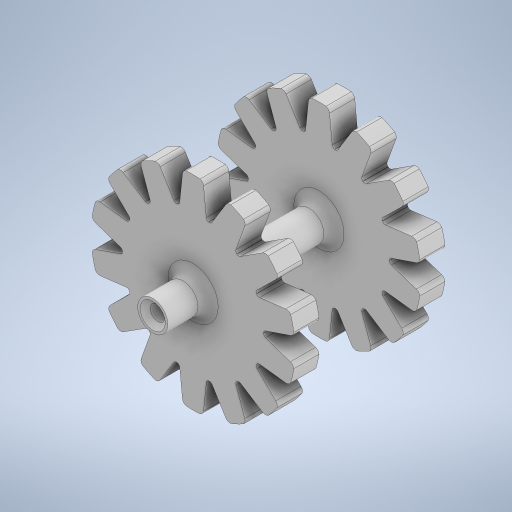
# Autodesk Inventor part: Zebatka
Saved by Autodesk Inventor 2024 (Build 280153000, 153)
## iProperties
Created: 2025-05-18
Part Number: Zebatka
Material: Ogólny
Document SubType Name: Modeling
Designer: Victoria
Density: 1 g/cm^3
Appearance: Domyślna
Author: Victoria
Autodesk Inventor part; units mm, degrees
ref_plane "YZ Plane" through (0, 0, 0) normal (1, 0, 0) x (0, 1, 0)
ref_plane "XZ Plane" through (0, 0, 0) normal (0, 1, 0) x (-1, 0, 0)
ref_plane "XY Plane" through (0, 0, 0) normal (0, 0, 1) x (1, 0, 0)
sketch "Szkic2" plane through (0, 0, 0) normal (0, 0, 1) x (1, 0, 0)
  circle A0 centre (0, 0) radius 20.25
  line L0 (0, 20.25) -> (1.0996, 20.25)
  line L1 (0, 20.25) -> (-1.0996, 20.25)
  circle A1 centre (0, 0) radius 14
  line L2 (-2.0941, 19.3545) -> (-2.6842, 13.7403)
  line L3 (-2, 20.25) -> (3.6452, 20.25) construction
  line L4 (2.0941, 19.3545) -> (2.6842, 13.7403)
  line L5 (2, 20.25) -> (7.6452, 20.25) construction
  arc A2 (-1.0996, 20.25) -> (-2.0941, 19.3545) centre (-1.0996, 19.25) ccw
  arc A3 (2.0941, 19.3545) -> (1.0996, 20.25) centre (1.0996, 19.25) ccw
  line L6 (-10.2844, 16.5292) -> (-8.3801, 11.2149)
  arc A4 (-9.7768, 17.7675) -> (-10.2844, 16.5292) centre (-9.343, 16.8666) ccw
  line L7 (-8.7861, 18.2446) -> (-9.7768, 17.7675)
  line L8 (-8.7861, 18.2446) -> (-7.7954, 18.7217)
  arc A5 (-6.5109, 18.3464) -> (-7.7954, 18.7217) centre (-7.3616, 17.8207) ccw
  line L9 (-6.5109, 18.3464) -> (-3.5433, 13.5442)
  line L10 (-16.4376, 10.4301) -> (-12.4161, 6.4683)
  arc A6 (-16.5177, 11.766) -> (-16.4376, 10.4301) centre (-15.7358, 11.1425) ccw
  line L11 (-15.8321, 12.6257) -> (-16.5177, 11.766)
  line L12 (-15.8321, 12.6257) -> (-15.1465, 13.4854)
  arc A7 (-13.8263, 13.7046) -> (-15.1465, 13.4854) centre (-14.3647, 12.8619) ccw
  line L13 (-13.8263, 13.7046) -> (-9.069, 10.6655)
  line L14 (-19.3353, 2.2652) -> (-13.9931, 0.4406)
  arc A8 (-19.987, 3.434) -> (-19.3353, 2.2652) centre (-19.012, 3.2115) ccw
  line L15 (-19.7423, 4.506) -> (-19.987, 3.434)
  line L16 (-19.7423, 4.506) -> (-19.4976, 5.5781)
  arc A9 (-18.4033, 6.3484) -> (-19.4976, 5.5781) centre (-18.5227, 5.3556) ccw
  line L17 (-18.4033, 6.3484) -> (-12.7985, 5.6744)
  line L18 (-18.4033, -6.3484) -> (-12.7985, -5.6744)
  arc A10 (-19.4976, -5.5781) -> (-18.4033, -6.3484) centre (-18.5227, -5.3556) ccw
  line L19 (-19.7423, -4.506) -> (-19.4976, -5.5781)
  line L20 (-19.7423, -4.506) -> (-19.987, -3.434)
  arc A11 (-19.3353, -2.2652) -> (-19.987, -3.434) centre (-19.012, -3.2115) ccw
  line L21 (-19.3353, -2.2652) -> (-13.9931, -0.4406)
  line L22 (-13.8263, -13.7046) -> (-9.069, -10.6655)
  arc A12 (-15.1465, -13.4854) -> (-13.8263, -13.7046) centre (-14.3647, -12.8619) ccw
  line L23 (-15.8321, -12.6257) -> (-15.1465, -13.4854)
  line L24 (-15.8321, -12.6257) -> (-16.5177, -11.766)
  arc A13 (-16.4376, -10.4301) -> (-16.5177, -11.766) centre (-15.7358, -11.1425) ccw
  line L25 (-16.4376, -10.4301) -> (-12.4161, -6.4683)
  line L26 (-6.5109, -18.3464) -> (-3.5433, -13.5442)
  arc A14 (-7.7954, -18.7217) -> (-6.5109, -18.3464) centre (-7.3616, -17.8207) ccw
  line L27 (-8.7861, -18.2446) -> (-7.7954, -18.7217)
  line L28 (-8.7861, -18.2446) -> (-9.7768, -17.7675)
  arc A15 (-10.2844, -16.5292) -> (-9.7768, -17.7675) centre (-9.343, -16.8666) ccw
  line L29 (-10.2844, -16.5292) -> (-8.3801, -11.2149)
  line L30 (2.0941, -19.3545) -> (2.6842, -13.7403)
  arc A16 (1.0996, -20.25) -> (2.0941, -19.3545) centre (1.0996, -19.25) ccw
  line L31 (0, -20.25) -> (1.0996, -20.25)
  line L32 (0, -20.25) -> (-1.0996, -20.25)
  arc A17 (-2.0941, -19.3545) -> (-1.0996, -20.25) centre (-1.0996, -19.25) ccw
  line L33 (-2.0941, -19.3545) -> (-2.6842, -13.7403)
  line L34 (10.2844, -16.5292) -> (8.3801, -11.2149)
  arc A18 (9.7768, -17.7675) -> (10.2844, -16.5292) centre (9.343, -16.8666) ccw
  line L35 (8.7861, -18.2446) -> (9.7768, -17.7675)
  line L36 (8.7861, -18.2446) -> (7.7954, -18.7217)
  arc A19 (6.5109, -18.3464) -> (7.7954, -18.7217) centre (7.3616, -17.8207) ccw
  line L37 (6.5109, -18.3464) -> (3.5433, -13.5442)
  line L38 (16.4376, -10.4301) -> (12.4161, -6.4683)
  arc A20 (16.5177, -11.766) -> (16.4376, -10.4301) centre (15.7358, -11.1425) ccw
  line L39 (15.8321, -12.6257) -> (16.5177, -11.766)
  line L40 (15.8321, -12.6257) -> (15.1465, -13.4854)
  arc A21 (13.8263, -13.7046) -> (15.1465, -13.4854) centre (14.3647, -12.8619) ccw
  line L41 (13.8263, -13.7046) -> (9.069, -10.6655)
  line L42 (19.3353, -2.2652) -> (13.9931, -0.4406)
  arc A22 (19.987, -3.434) -> (19.3353, -2.2652) centre (19.012, -3.2115) ccw
  line L43 (19.7423, -4.506) -> (19.987, -3.434)
  line L44 (19.7423, -4.506) -> (19.4976, -5.5781)
  arc A23 (18.4033, -6.3484) -> (19.4976, -5.5781) centre (18.5227, -5.3556) ccw
  line L45 (18.4033, -6.3484) -> (12.7985, -5.6744)
  line L46 (18.4033, 6.3484) -> (12.7985, 5.6744)
  arc A24 (19.4976, 5.5781) -> (18.4033, 6.3484) centre (18.5227, 5.3556) ccw
  line L47 (19.7423, 4.506) -> (19.4976, 5.5781)
  line L48 (19.7423, 4.506) -> (19.987, 3.434)
  arc A25 (19.3353, 2.2652) -> (19.987, 3.434) centre (19.012, 3.2115) ccw
  line L49 (19.3353, 2.2652) -> (13.9931, 0.4406)
  line L50 (13.8263, 13.7046) -> (9.069, 10.6655)
  arc A26 (15.1465, 13.4854) -> (13.8263, 13.7046) centre (14.3647, 12.8619) ccw
  line L51 (15.8321, 12.6257) -> (15.1465, 13.4854)
  line L52 (15.8321, 12.6257) -> (16.5177, 11.766)
  arc A27 (16.4376, 10.4301) -> (16.5177, 11.766) centre (15.7358, 11.1425) ccw
  line L53 (16.4376, 10.4301) -> (12.4161, 6.4683)
  line L54 (6.5109, 18.3464) -> (3.5433, 13.5442)
  arc A28 (7.7954, 18.7217) -> (6.5109, 18.3464) centre (7.3616, 17.8207) ccw
  line L55 (8.7861, 18.2446) -> (7.7954, 18.7217)
  line L56 (8.7861, 18.2446) -> (9.7768, 17.7675)
  arc A29 (10.2844, 16.5292) -> (9.7768, 17.7675) centre (9.343, 16.8666) ccw
  line L57 (10.2844, 16.5292) -> (8.3801, 11.2149)
  circle A30 centre (0, 0) radius 1.5
  point P0 (-10.5881, 17.3769)
  point P1 (-6.9842, 19.1124)
  point P2 (-17.0791, 11.062)
  point P3 (-14.5851, 14.1893)
  point P4 (-20.1873, 2.5562)
  point P5 (-19.2972, 6.4559)
  point P6 (-19.2972, -6.4559)
  point P7 (-20.1873, -2.5562)
  point P8 (-14.5851, -14.1893)
  point P9 (-17.0791, -11.062)
  point P10 (-6.9842, -19.1124)
  point P11 (-10.5881, -17.3769)
  point P12 (2, -20.25)
  point P13 (-2, -20.25)
  point P14 (10.5881, -17.3769)
  point P15 (6.9842, -19.1124)
  point P16 (17.0791, -11.062)
  point P17 (14.5851, -14.1893)
  point P18 (20.1873, -2.5562)
  point P19 (19.2972, -6.4559)
  point P20 (19.2972, 6.4559)
  point P21 (20.1873, 2.5562)
  point P22 (14.5851, 14.1893)
  point P23 (17.0791, 11.062)
  point P24 (6.9842, 19.1124)
  point P25 (10.5881, 17.3769)
  point P26 (-14.9152, 13.6967)
  point P27 (-16.6722, 11.4934)
  point P28 (-19.3809, 5.8688)
  point P29 (-20.008, 3.1214)
  point P30 (-20.008, -3.1214)
  point P31 (-19.3809, -5.8688)
  point P32 (-16.6722, -11.4934)
  point P33 (-14.9152, -13.6967)
  point P34 (-10.0343, -17.589)
  point P35 (-7.4954, -18.8118)
  point P36 (-1.409, -20.2009)
  point P37 (1.409, -20.2009)
  point P38 (7.4954, -18.8118)
  point P39 (10.0343, -17.589)
  point P40 (14.9152, -13.6967)
  point P41 (16.6722, -11.4934)
  point P42 (19.3809, -5.8688)
  point P43 (20.008, -3.1214)
  point P44 (20.008, 3.1214)
  point P45 (19.3809, 5.8688)
  point P46 (16.6722, 11.4934)
  point P47 (14.9152, 13.6967)
  point P48 (10.0343, 17.589)
  point P49 (7.4954, 18.8118)
  point P50 (1.409, 20.2009)
  point P51 (-1.409, 20.2009)
  point P52 (-7.4954, 18.8118)
  point P53 (-10.0343, 17.589)
  dimension "d14" = 40.5
  dimension "d17" = 6.25
  dimension "d15" = 2
  dimension "d16" = 2
  dimension "d18" = 264
  dimension "d19" = 84
  dimension "d20" = 1
  dimension "d23" = 360
  dimension "d25" = 3
  constraints: 116 end point, 70 point on line, 56 point on circle, 29 centre point, 4 horizontal, 4 tangent, 2 coincident, 2 equal length, 1 equal radius, 246 other
  measures "d15" distance of L0.start L5.start
  measures "d16" distance of L0.start L3.start
  measures "d19" angle of L4 L5
  measures "d20" radius of A2
  measures "d25" diameter of A30
extrude "Wyciągnięcie proste2" add sketch "Szkic2" along normal blind 5 contours A25 L49 A1 L46 A24 A0 | A0 A23 L45 A1 L42 A22 | A1 | A27 L53 A1 L50 A26 A0 | A0 A21 L41 A1 L38 A20 | A29 L57 A1 L54 A28 A0 | A0 A19 L37 A1 L34 A18 | A1 L2 A2 A0 A3 L4 | L30 A16 A0 A17 L33 A1 | A1 L6 A4 A0 A5 L9 | L26 A14 A0 A15 L29 A1 | A1 L10 A6 A0 A7 L13 | L22 A12 A0 A13 L25 A1 | A1 L14 A8 A0 A9 L17 | L18 A10 A0 A11 L21 A1
fillet "Zaokrąglenie1" radius 0.6 28 edges at (-13.9931, 0.4406, 2.5) (-13.9931, -0.4406, 2.5) (-12.7985, -5.6744, 2.5) (-12.4161, -6.4683, 2.5) (-8.3801, -11.2149, 2.5) (-9.069, -10.6655, 2.5) (-2.6842, -13.7403, 2.5) (-3.5433, -13.5442, 2.5) (3.5433, -13.5442, 2.5) (2.6842, -13.7403, 2.5) (9.069, -10.6655, 2.5) (8.3801, -11.2149, 2.5) (12.7985, -5.6744, 2.5) (12.4161, -6.4683, 2.5) (13.9931, 0.4406, 2.5) (13.9931, -0.4406, 2.5) (12.7985, 5.6744, 2.5) (12.4161, 6.4683, 2.5) (8.3801, 11.2149, 2.5) (9.069, 10.6655, 2.5) (2.6842, 13.7403, 2.5) (3.5433, 13.5442, 2.5) (-3.5433, 13.5442, 2.5) (-2.6842, 13.7403, 2.5) (-9.069, 10.6655, 2.5) (-8.3801, 11.2149, 2.5) (-12.7985, 5.6744, 2.5) (-12.4161, 6.4683, 2.5)
sketch "Szkic3" plane through (0, 0, 5) normal (0, 0, 1) x (1, 0, 0)
  circle A0 centre (0, 0) radius 1.5 projected
  circle A1 centre (0, 0) radius 3
  dimension "d29" = 6
  constraints: 1 centre point, 1 coincident
  measures "d29" diameter of A1
extrude "Wyciągnięcie proste3" add sketch "Szkic3" along normal blind 20 and the other way blind 8
sketch "Szkic4" plane through (0, 0, 25) normal (0, 0, 1) x (1, 0, 0)
  circle A0 centre (0, 0) radius 3 projected
  arc A1 (-13.8263, 13.7046) -> (-14.9152, 13.6967) centre (-14.3647, 12.8619) ccw projected
  arc A2 (-14.9152, 13.6967) -> (-16.6722, 11.4934) centre (0, 0) ccw projected
  arc A3 (-16.6722, 11.4934) -> (-16.4376, 10.4301) centre (-15.7358, 11.1425) ccw projected
  line L0 (-16.4376, 10.4301) -> (-12.727, 6.7746) projected
  arc A4 (-12.6078, 6.0863) -> (-12.727, 6.7746) centre (-13.1481, 6.3472) ccw projected
  arc A5 (-12.6078, 6.0863) -> (-12.6193, 6.0624) centre (0, 0) ccw projected
  arc A6 (-13.2318, 5.7265) -> (-12.6193, 6.0624) centre (-13.1602, 6.3222) ccw projected
  line L1 (-13.2318, 5.7265) -> (-18.4033, 6.3484) projected
  arc A7 (-18.4033, 6.3484) -> (-19.3809, 5.8688) centre (-18.5227, 5.3556) ccw projected
  arc A8 (-19.3809, 5.8688) -> (-20.008, 3.1214) centre (0, 0) ccw projected
  arc A9 (-20.008, 3.1214) -> (-19.3353, 2.2652) centre (-19.012, 3.2115) ccw projected
  line L2 (-19.3353, 2.2652) -> (-14.4061, 0.5817) projected
  arc A10 (-14, 0.0133) -> (-14.4061, 0.5817) centre (-14.6, 0.0139) ccw projected
  arc A11 (-14, 0.0133) -> (-14, -0.0133) centre (0, 0) ccw projected
  arc A12 (-14.4061, -0.5817) -> (-14, -0.0133) centre (-14.6, -0.0139) ccw projected
  line L3 (-14.4061, -0.5817) -> (-19.3353, -2.2652) projected
  arc A13 (-19.3353, -2.2652) -> (-20.008, -3.1214) centre (-19.012, -3.2115) ccw projected
  arc A14 (-20.008, -3.1214) -> (-19.3809, -5.8688) centre (0, 0) ccw projected
  arc A15 (-19.3809, -5.8688) -> (-18.4033, -6.3484) centre (-18.5227, -5.3556) ccw projected
  line L4 (-18.4033, -6.3484) -> (-13.2318, -5.7265) projected
  arc A16 (-12.6193, -6.0624) -> (-13.2318, -5.7265) centre (-13.1602, -6.3222) ccw projected
  arc A17 (-12.6193, -6.0624) -> (-12.6078, -6.0863) centre (0, 0) ccw projected
  arc A18 (-12.727, -6.7746) -> (-12.6078, -6.0863) centre (-13.1481, -6.3472) ccw projected
  line L5 (-12.727, -6.7746) -> (-16.4376, -10.4301) projected
  arc A19 (-16.4376, -10.4301) -> (-16.6722, -11.4934) centre (-15.7358, -11.1425) ccw projected
  arc A20 (-16.6722, -11.4934) -> (-14.9152, -13.6967) centre (0, 0) ccw projected
  arc A21 (-14.9152, -13.6967) -> (-13.8263, -13.7046) centre (-14.3647, -12.8619) ccw projected
  line L6 (-13.8263, -13.7046) -> (-9.4368, -10.9005) projected
  arc A22 (-8.7392, -10.9374) -> (-9.4368, -10.9005) centre (-9.1138, -11.4061) ccw projected
  arc A23 (-8.7392, -10.9374) -> (-8.7185, -10.9539) centre (0, 0) ccw projected
  arc A24 (-8.5273, -11.6258) -> (-8.7185, -10.9539) centre (-9.0921, -11.4234) ccw projected
  line L7 (-8.5273, -11.6258) -> (-10.2844, -16.5292) projected
  arc A25 (-10.2844, -16.5292) -> (-10.0343, -17.589) centre (-9.343, -16.8666) ccw projected
  arc A26 (-10.0343, -17.589) -> (-7.4954, -18.8118) centre (0, 0) ccw projected
  arc A27 (-7.4954, -18.8118) -> (-6.5109, -18.3464) centre (-7.3616, -17.8207) ccw projected
  line L8 (-6.5109, -18.3464) -> (-3.7727, -13.9154) projected
  arc A28 (-3.1282, -13.646) -> (-3.7727, -13.9154) centre (-3.2623, -14.2309) ccw projected
  arc A29 (-3.1282, -13.646) -> (-3.1023, -13.6519) centre (0, 0) ccw projected
  arc A30 (-2.6386, -14.1743) -> (-3.1023, -13.6519) centre (-3.2353, -14.237) ccw projected
  line L9 (-2.6386, -14.1743) -> (-2.0941, -19.3545) projected
  arc A31 (-2.0941, -19.3545) -> (-1.409, -20.2009) centre (-1.0996, -19.25) ccw projected
  arc A32 (-1.409, -20.2009) -> (1.409, -20.2009) centre (0, 0) ccw projected
  arc A33 (1.409, -20.2009) -> (2.0941, -19.3545) centre (1.0996, -19.25) ccw projected
  line L10 (2.0941, -19.3545) -> (2.6386, -14.1743) projected
  arc A34 (3.1023, -13.6519) -> (2.6386, -14.1743) centre (3.2353, -14.237) ccw projected
  arc A35 (3.1023, -13.6519) -> (3.1282, -13.646) centre (0, 0) ccw projected
  arc A36 (3.7727, -13.9154) -> (3.1282, -13.646) centre (3.2623, -14.2309) ccw projected
  line L11 (3.7727, -13.9154) -> (6.5109, -18.3464) projected
  arc A37 (6.5109, -18.3464) -> (7.4954, -18.8118) centre (7.3616, -17.8207) ccw projected
  arc A38 (7.4954, -18.8118) -> (10.0343, -17.589) centre (0, 0) ccw projected
  arc A39 (10.0343, -17.589) -> (10.2844, -16.5292) centre (9.343, -16.8666) ccw projected
  line L12 (10.2844, -16.5292) -> (8.5273, -11.6258) projected
  arc A40 (8.7185, -10.9539) -> (8.5273, -11.6258) centre (9.0921, -11.4234) ccw projected
  arc A41 (8.7185, -10.9539) -> (8.7392, -10.9374) centre (0, 0) ccw projected
  arc A42 (9.4368, -10.9005) -> (8.7392, -10.9374) centre (9.1138, -11.4061) ccw projected
  line L13 (9.4368, -10.9005) -> (13.8263, -13.7046) projected
  arc A43 (13.8263, -13.7046) -> (14.9152, -13.6967) centre (14.3647, -12.8619) ccw projected
  arc A44 (14.9152, -13.6967) -> (16.6722, -11.4934) centre (0, 0) ccw projected
  arc A45 (16.6722, -11.4934) -> (16.4376, -10.4301) centre (15.7358, -11.1425) ccw projected
  line L14 (16.4376, -10.4301) -> (12.727, -6.7746) projected
  arc A46 (12.6078, -6.0863) -> (12.727, -6.7746) centre (13.1481, -6.3472) ccw projected
  arc A47 (12.6078, -6.0863) -> (12.6193, -6.0624) centre (0, 0) ccw projected
  arc A48 (13.2318, -5.7265) -> (12.6193, -6.0624) centre (13.1602, -6.3222) ccw projected
  line L15 (13.2318, -5.7265) -> (18.4033, -6.3484) projected
  arc A49 (18.4033, -6.3484) -> (19.3809, -5.8688) centre (18.5227, -5.3556) ccw projected
  arc A50 (19.3809, -5.8688) -> (20.008, -3.1214) centre (0, 0) ccw projected
  arc A51 (20.008, -3.1214) -> (19.3353, -2.2652) centre (19.012, -3.2115) ccw projected
  line L16 (19.3353, -2.2652) -> (14.4061, -0.5817) projected
  arc A52 (14, -0.0133) -> (14.4061, -0.5817) centre (14.6, -0.0139) ccw projected
  arc A53 (14, -0.0133) -> (14, 0.0133) centre (0, 0) ccw projected
  arc A54 (14.4061, 0.5817) -> (14, 0.0133) centre (14.6, 0.0139) ccw projected
  line L17 (14.4061, 0.5817) -> (19.3353, 2.2652) projected
  arc A55 (19.3353, 2.2652) -> (20.008, 3.1214) centre (19.012, 3.2115) ccw projected
  arc A56 (20.008, 3.1214) -> (19.3809, 5.8688) centre (0, 0) ccw projected
  arc A57 (19.3809, 5.8688) -> (18.4033, 6.3484) centre (18.5227, 5.3556) ccw projected
  line L18 (18.4033, 6.3484) -> (13.2318, 5.7265) projected
  arc A58 (12.6193, 6.0624) -> (13.2318, 5.7265) centre (13.1602, 6.3222) ccw projected
  arc A59 (12.6193, 6.0624) -> (12.6078, 6.0863) centre (0, 0) ccw projected
  arc A60 (12.727, 6.7746) -> (12.6078, 6.0863) centre (13.1481, 6.3472) ccw projected
  line L19 (12.727, 6.7746) -> (16.4376, 10.4301) projected
  arc A61 (16.4376, 10.4301) -> (16.6722, 11.4934) centre (15.7358, 11.1425) ccw projected
  arc A62 (16.6722, 11.4934) -> (14.9152, 13.6967) centre (0, 0) ccw projected
  arc A63 (14.9152, 13.6967) -> (13.8263, 13.7046) centre (14.3647, 12.8619) ccw projected
  line L20 (13.8263, 13.7046) -> (9.4368, 10.9005) projected
  arc A64 (8.7392, 10.9374) -> (9.4368, 10.9005) centre (9.1138, 11.4061) ccw projected
  arc A65 (8.7392, 10.9374) -> (8.7185, 10.9539) centre (0, 0) ccw projected
  arc A66 (8.5273, 11.6258) -> (8.7185, 10.9539) centre (9.0921, 11.4234) ccw projected
  line L21 (8.5273, 11.6258) -> (10.2844, 16.5292) projected
  arc A67 (10.2844, 16.5292) -> (10.0343, 17.589) centre (9.343, 16.8666) ccw projected
  arc A68 (10.0343, 17.589) -> (7.4954, 18.8118) centre (0, 0) ccw projected
  arc A69 (7.4954, 18.8118) -> (6.5109, 18.3464) centre (7.3616, 17.8207) ccw projected
  line L22 (6.5109, 18.3464) -> (3.7727, 13.9154) projected
  arc A70 (3.1282, 13.646) -> (3.7727, 13.9154) centre (3.2623, 14.2309) ccw projected
  arc A71 (3.1282, 13.646) -> (3.1023, 13.6519) centre (0, 0) ccw projected
  arc A72 (2.6386, 14.1743) -> (3.1023, 13.6519) centre (3.2353, 14.237) ccw projected
  line L23 (2.6386, 14.1743) -> (2.0941, 19.3545) projected
  arc A73 (2.0941, 19.3545) -> (1.409, 20.2009) centre (1.0996, 19.25) ccw projected
  arc A74 (1.409, 20.2009) -> (-1.409, 20.2009) centre (0, 0) ccw projected
  arc A75 (-1.409, 20.2009) -> (-2.0941, 19.3545) centre (-1.0996, 19.25) ccw projected
  line L24 (-2.0941, 19.3545) -> (-2.6386, 14.1743) projected
  arc A76 (-3.1023, 13.6519) -> (-2.6386, 14.1743) centre (-3.2353, 14.237) ccw projected
  arc A77 (-3.1023, 13.6519) -> (-3.1282, 13.646) centre (0, 0) ccw projected
  arc A78 (-3.7727, 13.9154) -> (-3.1282, 13.646) centre (-3.2623, 14.2309) ccw projected
  line L25 (-3.7727, 13.9154) -> (-6.5109, 18.3464) projected
  arc A79 (-6.5109, 18.3464) -> (-7.4954, 18.8118) centre (-7.3616, 17.8207) ccw projected
  arc A80 (-7.4954, 18.8118) -> (-10.0343, 17.589) centre (0, 0) ccw projected
  arc A81 (-10.0343, 17.589) -> (-10.2844, 16.5292) centre (-9.343, 16.8666) ccw projected
  line L26 (-10.2844, 16.5292) -> (-8.5273, 11.6258) projected
  arc A82 (-8.7185, 10.9539) -> (-8.5273, 11.6258) centre (-9.0921, 11.4234) ccw projected
  arc A83 (-8.7185, 10.9539) -> (-8.7392, 10.9374) centre (0, 0) ccw projected
  arc A84 (-9.4368, 10.9005) -> (-8.7392, 10.9374) centre (-9.1138, 11.4061) ccw projected
  line L27 (-9.4368, 10.9005) -> (-13.8263, 13.7046) projected
  circle A85 centre (0, 0) radius 3 projected
  circle A86 centre (0, 0) radius 1.5 projected
extrude "Wyciągnięcie proste4" add sketch "Szkic4" along normal blind 5 contours A0 | L27 A84 A83 A82 L26 A81 A80 A79 L25 A78 A77 A76 L24 A75 A74 A73 L23 A72 A71 A70 L22 A69 A68 A67 L21 A66 A65 A64 L20 A63 A62 A61 L19 A60 A59 A58 L18 A57 A56 A55 L17 A54 A53 A52 L16 A51 A50 A49 L15 A48 A47 A46 L14 A45 A44 A43 L13 A42 A41 A40 L12 A39 A38 A37 L11 A36 A35 A34 L10 A33 A32 A31 L9 A30 A29 A28 L8 A27 A26 A25 L7 A24 A23 A22 L6 A21 A20 A19 L5 A18 A17 A16 L4 A15 A14 A13 L3 A12 A11 A10 L2 A9 A8 A7 L1 A6 A5 A4 L0 A3 A2 A1
sketch "Szkic5" plane through (0, 0, 30) normal (0, 0, 1) x (1, 0, 0)
  circle A0 centre (0, 0) radius 3 projected
  circle A1 centre (0, 0) radius 1.5 projected
extrude "Wyciągnięcie proste5" add sketch "Szkic5" along normal blind 8
fillet "Zaokrąglenie2" radius 2 4 edges at (-3, 0, 30) (-3, 0, 25) (-3, 0, 0) (-3, 0, 5)
chamfer "Faza1" distance 1 angle 45 2 edges at (-1.5, 0, -3) (-1.5, 0, 38)
